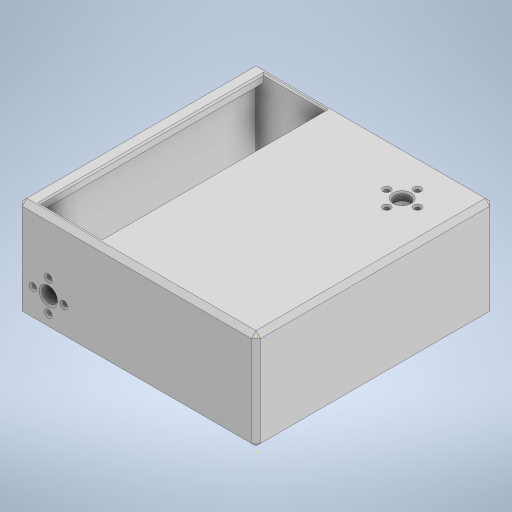
# Autodesk Inventor part: Water container
Saved by Autodesk Inventor 2023 (Build 270158000, 158)
## iProperties
Created: 2022-11-25
Part Number: Water container
Material: Generic
Document SubType Name: Sheet Metal
Designer: hp
Density: 1 g/cm^3
Sheet Metal Rule: Default_mm
Appearance: Default
Author: hp
Autodesk Inventor part; units mm, degrees
ref_plane "YZ Plane" through (0, 0, 0) normal (1, 0, 0) x (0, 1, 0)
ref_plane "XZ Plane" through (0, 0, 0) normal (0, 1, 0) x (-1, 0, 0)
ref_plane "XY Plane" through (0, 0, 0) normal (0, 0, 1) x (1, 0, 0)
sketch "Sketch1" plane through (0, 0, 0) normal (0, 1, 0) x (-1, 0, 0)
  line L0 (0, 0) -> (155, 0)
  line L1 (155, 0) -> (155, -155)
  line L2 (155, -155) -> (0, -155)
  line L3 (0, -155) -> (0, 0)
  dimension "d0" = 155
  dimension "d1" = 155
  constraints: 8 end point, 2 parallel, 1 horizontal, 1 perpendicular
  measures "d0" distance of L2.end L0.start
  measures "d1" distance of L1.end L2.end
extrude "Extrusion1" add sketch "Sketch1" along normal blind 60
sketch "Sketch2" plane through (0, 60, 0) normal (0, 1, 0) x (1, 0, 0)
  line L0 (-150, 5) -> (-5, 5)
  line L1 (-5, 5) -> (-5, 150)
  line L2 (-5, 150) -> (-150, 150)
  line L3 (-150, 150) -> (-150, 5)
  line L4 (-155, 0) -> (0, 0) projected
  line L5 (0, 155) -> (-155, 155) projected
  line L6 (-155, 155) -> (-155, 0) projected
  line L7 (0, 0) -> (0, 155) projected
  point P0 (-77.5, 155)
  dimension "d4" = 5
  dimension "d5" = 5
  dimension "d6" = 5
  dimension "d7" = 5
  constraints: 8 end point, 2 parallel, 1 horizontal, 1 midpoint, 1 perpendicular
  measures "d4" distance between parallel lines of L4 L0
  measures "d5" distance from line of point (-77.5, 155) L2
  measures "d6" distance between parallel lines of L6 L3
  measures "d7" distance between parallel lines of L7 L1
extrude "Extrusion2" cut sketch "Sketch2" against normal blind 55 contours L3 L2 L1 L0
sketch "Sketch3" plane through (0, 60, 0) normal (0, 1, 0) x (1, 0, 0)
  line L0 (-155, 0) -> (0, 0) projected
  line L1 (-155, 0) -> (0, 0)
  line L2 (0, 0) -> (0, 155)
  line L3 (0, 155) -> (-155, 155)
  line L4 (-155, 155) -> (-155, 0)
  constraints: 8 end point, 2 parallel, 1 horizontal, 1 perpendicular
extrude "Extrusion3" add sketch "Sketch3" along normal blind 5
sketch "Sketch4" plane through (0, 65, 0) normal (0, 1, 0) x (1, 0, 0)
  circle A0 centre (-30, 125) radius 5
  line L0 (0, 155) -> (-155, 155) projected
  line L1 (0, 0) -> (0, 155) projected
  dimension "d12" = 10
  dimension "d13" = 30
  dimension "d14" = 30
  constraints: 1 centre point
  measures "d12" diameter of A0
  measures "d13" distance from line of L0 A0.centre
  measures "d14" distance from line of L1 A0.centre
extrude "Extrusion4" cut sketch "Sketch4" against normal blind 5
sketch "Sketch5" plane through (-155, 0, 0) normal (0, 0, 1) x (1, 0, 0)
  circle A0 centre (20, 20) radius 5
  line L0 (0, 0) -> (155, 0) projected
  line L1 (0, 0) -> (0, 65) projected
  dimension "d17" = 20
  dimension "d18" = 20
  dimension "d19" = 10
  constraints: 1 centre point
  measures "d17" distance from line of L0 A0.centre
  measures "d18" distance from line of L1 A0.centre
  measures "d19" diameter of A0
extrude "Extrusion5" cut sketch "Sketch5" against normal blind 20
sketch "Sketch6" plane through (0, 65, 0) normal (0, 1, 0) x (1, 0, 0)
  line L0 (-145, 5) -> (-105, 5)
  line L1 (-105, 5) -> (-105, 150)
  line L2 (-105, 150) -> (-145, 150)
  line L3 (-145, 150) -> (-145, 5)
  line L4 (-155, 155) -> (-155, 0) projected
  line L5 (0, 155) -> (-155, 155) projected
  line L6 (-155, 0) -> (0, 0) projected
  point P0 (-125, 5)
  dimension "d22" = 10
  dimension "d23" = 5
  dimension "d24" = 5
  dimension "d25" = 40
  constraints: 8 end point, 2 parallel, 1 horizontal, 1 midpoint, 1 perpendicular
  measures "d22" distance between parallel lines of L4 L3
  measures "d23" distance between parallel lines of L5 L2
  measures "d24" distance from line of L6 point (-125, 5)
  measures "d25" distance between parallel lines of L3 L1
extrude "Extrusion6" cut sketch "Sketch6" against normal blind 5
sketch "Sketch7" plane through (-155, 0, 0) normal (0, 0, 1) x (1, 0, 0)
  circle A0 centre (20, 30) radius 1.5
  circle A1 centre (20, 20) radius 5 projected
  circle A2 centre (20, 20) radius 5
  circle A3 centre (10, 20) radius 1.5
  circle A4 centre (20, 10) radius 1.5
  circle A5 centre (30, 20) radius 1.5
  point P0 (155, 0)
  dimension "d28" = 3
  dimension "d31" = 360
  dimension "d35" = 10
  constraints: 5 centre point, 1 coincident, 9 other
  measures "d28" diameter of A0
  measures "d35" distance of A2.centre A0.centre
extrude "Extrusion7" cut sketch "Sketch7" against normal blind 5 contours A0 | A3 | A4 | A5
sketch "Sketch8" plane through (0, 65, 0) normal (0, 1, 0) x (1, 0, 0)
  point P0 (0, 0)
sketch "Sketch9" plane through (0, 65, 0) normal (0, 1, 0) x (1, 0, 0)
  point P0 (0, 0)
sketch "Sketch10" plane through (0, 65, 0) normal (0, 1, 0) x (1, 0, 0)
  point P0 (0, 0)
chamfer "Chamfer1" distance 1 angle 45 4 edges at (-126.5, 20, 0) (-136.5, 30, 0) (-136.5, 10, 0) (-146.5, 20, 0)
chamfer "Chamfer3" distance 1 angle 45 4 edges at (-105, 65, -77.5) (-125, 65, -150) (-145, 65, -77.5) (-125, 65, -5)
sketch "Sketch12" plane through (-5, 5, -5) normal (0, 0, -1) x (-1, 0, 0)
  line L0 (0, 0) -> (145, 0) projected
  line L1 (145, 0) -> (115, 0)
  line L2 (115, 0) -> (115, 30)
  line L3 (115, 30) -> (145, 30)
  line L4 (145, 30) -> (145, 0)
  point P0 (-5, -5)
  point P1 (115, 0)
  dimension "d53" = 30
  dimension "d54" = 30
  constraints: 8 end point, 2 parallel, 1 horizontal, 1 perpendicular
  measures "d53" distance of L2.end L3.end
  measures "d54" distance of L1.end L2.end
extrude "Extrusion9" add sketch "Sketch12" along normal blind 5
sketch "Sketch13" plane through (-155, 0, 0) normal (0, 0, 1) x (1, 0, 0)
  point P0 (155, 0)
sketch "Sketch14" plane through (-135, 20, -5) normal (0, 0, 1) x (1, 0, 0)
  circle A0 centre (0, 0) radius 5
  point P0 (135, -20)
  constraints: 1 centre point
extrude "Extrusion10" cut sketch "Sketch14" against normal blind 20
chamfer "Chamfer4" distance 1 angle 45 2 edges at (-35, 65, -125) (-140, 20, 0)
chamfer "Chamfer5" distance 3 angle 45 12 edges at (0, 65, -77.5) (-77.5, 65, 0) (-155, 65, -77.5) (-77.5, 65, -155) (0, 32.5, 0) (0, 32.5, -155) (-155, 32.5, -155) (-155, 32.5, 0) (0, 0, -77.5) (-77.5, 0, -155) (-155, 0, -77.5) (-77.5, 0, 0)
sketch "Sketch15" plane through (0, 65, 0) normal (0, 1, 0) x (1, 0, 0)
  point P0 (0, 0)
sketch "Sketch16" plane through (0, 65, 0) normal (0, 1, 0) x (1, 0, 0)
  point P0 (0, 0)
sketch "Sketch17" plane through (-152, 3, 0) normal (0, 0, 1) x (1, 0, 0)
  point P0 (152, -3)
sketch "Sketch18" plane through (-152, 3, 0) normal (0, 0, 1) x (1, 0, 0)
  point P0 (152, -3)
sketch "Sketch19" plane through (-152, 3, 0) normal (0, 0, 1) x (1, 0, 0)
  point P0 (152, -3)
sketch "Sketch20" plane through (0, 65, 0) normal (0, 1, 0) x (1, 0, 0)
  point P0 (0, 0)
sketch "Sketch21" plane through (-152, 3, 0) normal (0, 0, 1) x (1, 0, 0)
  point P0 (152, -3)
sketch "Sketch22" plane through (0, 65, 0) normal (0, 1, 0) x (1, 0, 0)
  circle A0 centre (-30, 135) radius 1.5
  circle A1 centre (-30, 125) radius 5 projected
  circle A2 centre (-40, 125) radius 1.5
  circle A3 centre (-30, 115) radius 1.5
  circle A4 centre (-20, 125) radius 1.5
  point P0 (0, 0)
  dimension "d66" = 3
  dimension "d67" = 10
  dimension "d70" = 360
  constraints: 4 centre point, 9 other
  measures "d66" diameter of A0
  measures "d67" distance of A1.centre A0.centre
sketch "Sketch23" plane through (-152, 3, 0) normal (0, 0, 1) x (1, 0, 0)
  point P0 (152, -3)
extrude "Extrusion11" cut sketch "Sketch22" against normal blind 10 contours A0 | A2 | A3 | A4
chamfer "Chamfer6" distance 1 angle 45 4 edges at (-21.5, 65, -125) (-31.5, 65, -135) (-41.5, 65, -125) (-31.5, 65, -115)
sketch "Sketch24" plane through (-152, 3, 0) normal (0, 0, 1) x (1, 0, 0)
  point P0 (152, -3)
equation "\"BendRadius\" = Thickness"
equation "\"BendReliefWidth\" = Thickness"
equation "\"BendReliefDepth\" = 0.5 * Thickness"
equation "\"CornerReliefSize\" = 4 * Thickness"
equation "\"MinimumRemnant\" = 2 * Thickness"
equation "\"TransitionRadius\" = BendRadius"
equation "\"JacobiRadiusSize\" = BendRadius"
equation "\"GapSize\" = Thickness"
equation "\"Thickness\" = 0.5"
body "Solid1"
